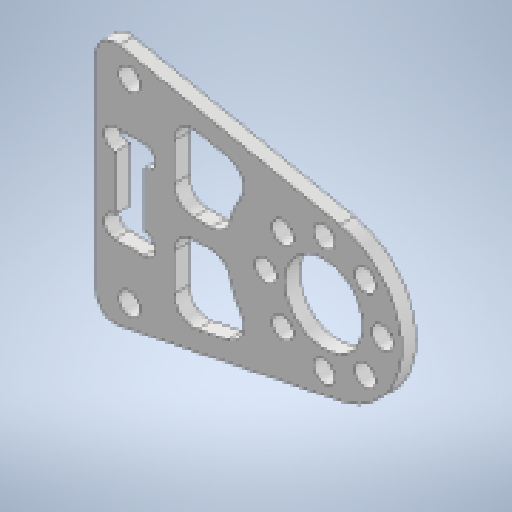
# Autodesk Inventor part: kata_new_1.5
Saved by Autodesk Inventor 2024 (Build 280153000, 153)
## iProperties
Created: 2023-12-16
Part Number: kata_new_1.5
Material: アルミニウム 2014-T4
Document SubType Name: Modeling
Designer: right
Density: 2.8 g/cm^3
Appearance: サテン
Mass: 1.58824 g
Surface Area: 11.6344 cm^2
Volume: 0.567228 cm^3
Author: right
Autodesk Inventor part; units mm, degrees
ref_plane "YZ Plane" through (0, 0, 0) normal (1, 0, 0) x (0, 1, 0)
ref_plane "XZ Plane" through (0, 0, 0) normal (0, 1, 0) x (-1, 0, 0)
ref_plane "XY Plane" through (0, 0, 0) normal (0, 0, 1) x (1, 0, 0)
sketch "スケッチ1" plane through (0, 0, 0) normal (0, 0, 1) x (1, 0, 0)
  circle A0 centre (1.5, 29.75) radius 0.7835 projected
  circle A1 centre (1.5, 9.75) radius 0.7835 projected
  line L0 (3, 24.75) -> (3, 14.75) projected
  line L1 (0, 24.75) -> (0, 14.75) projected
  line L2 (3, 24.75) -> (0, 24.75) projected
  line L3 (3, 14.75) -> (0, 14.75) projected
  circle A2 centre (3, 23.65) radius 1.1
  line L4 (3, 19.75) -> (0, 19.75) construction
  line L5 (1.5, 19.75) -> (1.5, 24.75) construction
  circle A3 centre (0, 23.65) radius 1.1
  line L6 (3, 14.75) -> (0, 14.75)
  circle A4 centre (3, 15.85) radius 1.1
  circle A5 centre (0, 15.85) radius 1.1
  circle A6 centre (1.5, 29.75) radius 1.1
  circle A7 centre (1.5, 9.75) radius 1.1
  line L7 (5.9977, 32.75) -> (-2, 32.75) construction
  line L8 (-2, 32.75) -> (-2, 6.75)
  line L9 (-2, 6.75) -> (5.9977, 6.75) construction
  line L10 (5.9977, 6.75) -> (5.9977, 32.75) construction
  line L11 (3, 32.75) -> (0, 32.75) projected
  line L12 (0, 6.75) -> (3, 6.75) projected
  circle A8 centre (21.5, 19.75) radius 4
  circle A9 centre (27.5, 19.75) radius 1.1
  circle A10 centre (25.7426, 23.9926) radius 1.1
  circle A11 centre (21.5, 25.75) radius 1.1
  circle A12 centre (17.2574, 23.9926) radius 1.1
  circle A13 centre (15.5, 19.75) radius 1.1
  circle A14 centre (17.2574, 15.5074) radius 1.1
  circle A15 centre (21.5, 13.75) radius 1.1
  circle A16 centre (25.7426, 15.5074) radius 1.1
  circle A17 centre (21.5, 19.75) radius 8
  line L13 (23.1114, 27.586) -> (-2, 32.75)
  line L14 (23.1114, 11.914) -> (-2, 6.75)
  point P0 (0, 0)
  point P1 (1.5, 14.75)
  point P2 (0, 16.95)
  point P3 (0, 22.55)
  point P4 (3, 22.55)
  point P5 (3, 16.95)
  dimension "d0" = 2.2
  dimension "d12" = 16
  dimension "d1" = 2.2
  dimension "d2" = 2
  dimension "d3" = 8
  dimension "d4" = 13
  dimension "d5" = 20
  dimension "d6" = 2.2
  dimension "d7" = 6
  dimension "d10" = 360
  constraints: 18 end point, 13 centre point, 6 symmetric about line, 4 midpoint, 3 horizontal alignment, 2 coincident, 2 horizontal, 2 parallel, 1 perpendicular, 1 point on line, 30 other
  measures "d1" diameter of A6
  measures "d2" distance from line of L8 A3.centre
  measures "d3" diameter of A8
  measures "d4" vertical distance of L8.end A8.centre
  measures "d5" distance of L5.start A8.centre
  measures "d6" diameter of A9
  measures "d7" distance of A8.centre A9.centre
extrude "押し出し1" add sketch "スケッチ1" along normal blind 1.5 contours L13 A17 L14 L8 | A17
fillet "フィレット1" radius 2 2 edges at (-2, 32.75, 0.75) (-2, 6.75, 0.75)
sketch "スケッチ2" plane through (0, 0, 0) normal (0, 0, -1) x (-1, 0, 0)
  circle A0 centre (-21.5, 19.75) radius 4 projected
  circle A1 centre (-21.5, 19.75) radius 8
  line L0 (-23.1114, 27.586) -> (-0.4029, 32.2559) projected
  line L1 (-6.1, 31.0843) -> (-6.1, 8.4157)
  arc A2 (-3, 24.75) -> (-3, 22.55) centre (-3, 23.65) ccw projected
  line L2 (-0.4029, 7.2441) -> (-23.1114, 11.914) projected
  circle A3 centre (-21.5, 19.75) radius 10
  line L3 (-14.8725, 27.2384) -> (-6.1, 29.0424)
  line L4 (-6.1, 19.75) -> (-11.5, 19.75) construction
  line L5 (-14.8725, 12.2616) -> (-6.1, 10.4576)
  line L6 (-6.0499, 18.75) -> (-11.5501, 18.75)
  line L7 (-11.5501, 18.75) -> (-11.5501, 20.75)
  line L8 (-11.5501, 20.75) -> (-6.0499, 20.75)
  line L9 (-6.0499, 20.75) -> (-6.0499, 18.75)
  line L10 (-6.0499, 18.75) -> (-11.5501, 20.75) construction
  line L11 (-11.5501, 18.75) -> (-6.0499, 20.75) construction
  point P0 (0, 0)
  point P1 (-4.1, 23.65)
  point P2 (-8.8, 19.75)
  point P3 (-6.1, 18.75)
  point P4 (-6.1, 20.75)
  dimension "d16" = 2
  dimension "d17" = 2
  dimension "d18" = 2
  dimension "d22" = 2
  constraints: 20 end point, 4 midpoint, 4 parallel, 4 point on circle, 3 point on line, 2 centre point, 2 symmetric about line, 1 coincident, 1 horizontal, 1 perpendicular, 1 tangent, 1 vertical
  measures "d16" distance from line of point (-4.1, 23.65) L1
  measures "d17" radial gap between concentric circles of A1 A3
  measures "d18" distance between parallel lines of L0 L3
  measures "d22" distance of L6.end L7.end
extrude "押し出し2" cut sketch "スケッチ2" against normal blind 1.5 contours L3 L1 L8 A3 | A3 L6 L1 L5
fillet "フィレット2" radius 2 8 edges at (14.8725, 27.2384, 0.75) (14.8725, 12.2616, 0.75) (6.1, 10.4576, 0.75) (6.1, 29.0424, 0.75) (11.5501, 20.75, 0.75) (6.1, 20.75, 0.75) (6.1, 18.75, 0.75) (11.5501, 18.75, 0.75)
equation "\"d18\" = d17"
